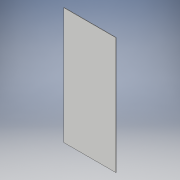
# Autodesk Inventor part: Ball Retainer Polycarb 19 x 8 5
Saved by Autodesk Inventor 2018 (Build 220112000, 112)
## iProperties
Created: 2020-01-31
Part Number: Ball Retainer Polycarb 19 x 8 5
Material: Generic
Document SubType Name: Modeling
Designer: Weeb No1
Density: 1 g/cm^3
Appearance: Default
Author: Weeb No1
Autodesk Inventor part; units mm, degrees
ref_plane "YZ Plane" through (0, 0, 0) normal (1, 0, 0) x (0, 1, 0)
ref_plane "XZ Plane" through (0, 0, 0) normal (0, 1, 0) x (-1, 0, 0)
ref_plane "XY Plane" through (0, 0, 0) normal (0, 0, 1) x (1, 0, 0)
sketch "Sketch1" plane through (0, 0, 0) normal (0, 0, 1) x (1, 0, 0)
  line L0 (0, 0) -> (215.9, 0)
  line L1 (215.9, 0) -> (215.9, 482.6)
  line L2 (215.9, 482.6) -> (0, 482.6)
  line L3 (0, 482.6) -> (0, 0)
  dimension "d0" = 215.9
  dimension "d1" = 482.6
  constraints: 8 end point, 2 parallel, 1 horizontal, 1 perpendicular
  measures "d0" distance of L2.end L1.end
  measures "d1" distance of L1.end L0.end
extrude "Extrusion1" add sketch "Sketch1" along normal blind 1.5875
body "Solid1"
